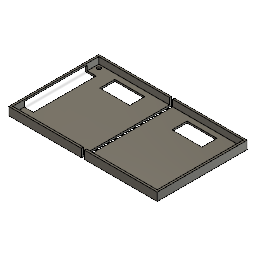
Screen_Case (Autodesk Fusion 360 design; units mm, degrees)
Autodesk Fusion 360 part; units mm, degrees
sketch "Sketch1" plane through (0, 0, 0) normal (0, 1, 0) x (1, 0, 0)
  line L0 (-122, 75.5) -> (122, 75.5)
  line L1 (122, 75.5) -> (122, -75.5)
  line L2 (122, -75.5) -> (-122, -75.5)
  line L3 (-122, -75.5) -> (-122, 75.5)
  line L4 (-122, 75.5) -> (122, -75.5) construction
  line L5 (122, 75.5) -> (-122, -75.5) construction
  dimension "d1" = 244
  dimension "d2" = 151
  constraint horizontal L0
  constraint perpendicular L0 L1
  constraint parallel L0 L2
  constraint parallel L1 L3
  constraint coincident L4 origin
  constraint coincident L5 origin
  measures "d1" distance of L1.end L2.end
  measures "d2" distance of L0.end L1.end
extrude "Extrude1" add sketch "Sketch1" along normal blind 14 makes body 1
sketch "Sketch3" plane through (0, 14, 0) normal (0, 1, 0) x (-1, 0, 0)
  line L0 (122, 75.5) -> (-122, 75.5)
  line L1 (-122, 75.5) -> (-122, -75.5)
  line L2 (-122, -75.5) -> (122, -75.5)
  line L3 (122, -75.5) -> (122, 75.5)
  line L4 (118.75, 72.25) -> (-118.75, 72.25)
  line L5 (-118.75, 72.25) -> (-118.75, -72.25)
  line L6 (-118.75, -72.25) -> (118.75, -72.25)
  line L7 (118.75, -72.25) -> (118.75, 72.25)
  line L8 (118.75, 72.25) -> (-118.75, -72.25) construction
  line L9 (-118.75, 72.25) -> (118.75, -72.25) construction
  dimension "d5" = 237.5
  dimension "d6" = 144.5
  constraint horizontal L4
  constraint perpendicular L4 L5
  constraint parallel L4 L6
  constraint parallel L5 L7
  constraint coincident L8 origin
  constraint coincident L9 origin
  measures "d5" distance of L5.end L6.end
  measures "d6" distance of L4.end L5.end
extrude "Extrude2" cut sketch "Sketch3" against normal blind 11 contours L4 L5 L6 L7 bodies 1
sketch "Sketch5" plane through (0, 5, 0) normal (0, 1, 0) x (-1, 0, 0)
  line L0 (118, -71.5) -> (118, 71.5)
  line L1 (118, 71.5) -> (-118, 71.5)
  line L2 (-118, 71.5) -> (-118, -71.5)
  line L3 (-118, -71.5) -> (118, -71.5)
  line L4 (0, 40.5) -> (-42, 40.5)
  line L5 (-42, 40.5) -> (48, 40.5)
  line L6 (48, 40.5) -> (48, -17.5)
  line L7 (48, -17.5) -> (-42, -17.5)
  line L8 (-42, -17.5) -> (-42, 40.5)
  constraint perpendicular L5 L6
  constraint perpendicular L6 L7
  constraint perpendicular L5 L8
extrude "Extrude3" [suppressed]
sketch "Sketch6" plane through (0, 3, 0) normal (0, 1, 0) x (-1, 0, 0)
  line L0 (118.75, -72.25) -> (118.75, 72.25)
  line L1 (118.75, 72.25) -> (-118.75, 72.25)
  line L2 (-118.75, 72.25) -> (-118.75, -72.25)
  line L3 (-118.75, -72.25) -> (118.75, -72.25)
  line L4 (118.75, -72.25) -> (123.75, -72.25) construction
  circle A0 centre (113, -66.5) radius 3.5
  circle A1 centre (113, 66.5) radius 3.5
  circle A2 centre (-113, 66.5) radius 3.5
  circle A3 centre (-113, -66.5) radius 3.5
  dimension "d18" = 7
  dimension "d21" = 7
  dimension "d22" = 7
  dimension "d23" = 7
  constraint horizontal L4
  constraint coincident L0.start L3.end
  measures "d18" diameter of A0
  measures "d21" diameter of A1
  measures "d22" diameter of A2
  measures "d23" diameter of A3
hole "Hole1" at (113, 3, -66.5) at (-113, 3, -66.5) at (-113, 3, 66.5) at (113, 3, 66.5) direction (0, -1, 0) diameter 6 depth 5 tip angle 180 bodies 1
sketch "Sketch7" plane through (0, 3, 0) normal (0, 1, 0) x (-1, 0, 0)
  circle A0 centre (113, 66.5) radius 3
  circle A1 centre (-113, -66.5) radius 3
  circle A2 centre (113, -66.5) radius 3
  circle A3 centre (-113, 66.5) radius 3
  line L0 (118.75, -72.25) -> (118.75, 72.25)
  line L1 (118.75, 72.25) -> (-118.75, 72.25)
  line L2 (-118.75, 72.25) -> (-118.75, -72.25)
  line L3 (-118.75, -72.25) -> (118.75, -72.25)
  line L4 (78, -63.5) -> (38, -63.5)
  line L5 (78, -63.5) -> (78, -45.5)
  line L6 (78, -45.5) -> (38, -45.5)
  line L7 (38, -45.5) -> (38, -63.5)
  line L8 (-78, -63.5) -> (-78, -45.5)
  line L9 (-78, -45.5) -> (-38, -45.5)
  line L10 (-38, -45.5) -> (-38, -63.5)
  line L11 (-38, -63.5) -> (-78, -63.5)
  line L12 (-38, -63.5) -> (-83, -63.5)
  line L13 (-83, -63.5) -> (-33, -63.5)
  line L14 (-33, -63.5) -> (-33, -38.5)
  line L15 (-33, -38.5) -> (-83, -38.5)
  line L16 (-83, -38.5) -> (-83, -63.5)
  line L17 (38, -63.5) -> (33, -63.5)
  line L18 (33, -63.5) -> (33, -38.5)
  line L19 (33, -38.5) -> (83, -38.5)
  line L20 (83, -38.5) -> (83, -63.5)
  line L21 (83, -63.5) -> (77.0132, -63.5)
  dimension "d37" = 45
  dimension "d38" = 50
  dimension "d39" = 25
  dimension "d40" = 5
  dimension "d41" = 50
  constraint perpendicular L0 L4
  constraint perpendicular L4 L5
  constraint perpendicular L5 L6
  constraint perpendicular L4 L7
  constraint perpendicular L6 L8
  constraint perpendicular L7 L9
  constraint perpendicular L4 L10
  constraint perpendicular L8 L11
  constraint perpendicular L8 L12
  constraint parallel L11 L13
  constraint perpendicular L13 L14
  constraint perpendicular L14 L15
  constraint perpendicular L13 L16
  constraint perpendicular L7 L17
  constraint perpendicular L15 L18
  constraint perpendicular L18 L19
  constraint perpendicular L19 L20
  constraint coincident L4 L21.end
  constraint perpendicular L5 L21
  measures "d37" distance of L10.end L12.end
  measures "d38" distance of L12.end L13.end
  measures "d39" distance of L13.end L14.end
  measures "d40" distance of L4.end L17.end
  measures "d41" distance of L18.end L19.end
extrude "Extrude4" cut sketch "Sketch7" against normal blind 20 contours L4 L5 L6 L7 L21 | L5 L6 L7 L17 L18 L19 L20 L21 | L8 L9 L10 L12 L13 L14 L15 L16 | L8 L9 L10 L11 L12 L13 bodies 1
split "Split1" by plane through (0, 0, 0) normal (1, 0, 0) bodies 1 makes body 2 at (47.8006, 0, 34)
move_body "Move1" bodies 2 to x (1, 0, 0) y (0, 1, 0) z (0, 0, 1) at (5, 0, 0)
sketch "Sketch8" plane through (0, 3, 0) normal (0, 1, 0) x (-1, 0, 0)
  line L0 (0, 72.25) -> (0, -72.25)
  line L1 (0, -72.25) -> (118.75, -72.25)
  line L2 (118.75, -72.25) -> (118.75, 72.25)
  line L3 (118.75, 72.25) -> (0, 72.25)
  line L4 (33, -38.5) -> (83, -38.5)
  line L5 (83, -38.5) -> (83, -63.5)
  line L6 (83, -63.5) -> (33, -63.5)
  line L7 (33, -63.5) -> (33, -38.5)
  circle A0 centre (113, 66.5) radius 3
  circle A1 centre (113, -66.5) radius 3
  line L8 (118.75, 72.25) -> (118.75, 52.25)
  line L9 (118.75, 52.25) -> (103.75, 52.25)
  line L10 (103.75, 52.25) -> (103.75, -52.75)
  line L11 (103.75, -52.75) -> (118.75, -52.75)
  line L12 (118.75, -52.75) -> (118.75, 52.25)
  dimension "d42" = 20
  dimension "d43" = 15
  dimension "d44" = 105
  constraint coincident L2.end L3.start
  constraint perpendicular L3 L8
  constraint horizontal L9
  constraint vertical L10
  constraint horizontal L11
  constraint vertical L12
  measures "d42" distance of L2.end L8.end
  measures "d43" distance of L8.end L9.end
  measures "d44" distance of L8.end L11.end
sketch "Sketch9" plane through (-118.75, 0, 0) normal (1, 0, 0) x (0, 0, -1)
  line L0 (72.25, 14) -> (-72.25, 14)
  line L1 (-72.25, 14) -> (-72.25, 3)
  line L2 (-72.25, 3) -> (72.25, 3)
  line L3 (72.25, 3) -> (72.25, 14)
  line L4 (52.75, 3) -> (-52.25, 3)
  line L5 (-52.25, 3) -> (-52.25, 11)
  line L6 (-52.25, 11) -> (52.75, 11)
  line L7 (52.75, 11) -> (52.75, 3)
  point P0 (52.75, 3)
  dimension "d45" = 8
  constraint horizontal L4
  constraint vertical L5
  constraint horizontal L6
  constraint vertical L7
  constraint coincident P0 L4.start
  measures "d45" distance of P0 L6.end
extrude "Extrude5" cut sketch "Sketch9" against normal blind 10 contours L2 L4 L5 L6 L7 bodies 1
extrude "Extrude6" cut sketch "Sketch8" against normal blind 20 contours L2 L9 L10 L11 L12 bodies 1
sketch "Sketch10" plane through (0, 3, 0) normal (0, 1, 0) x (-1, 0, 0)
  line L0 (118.75, 52.25) -> (118.75, -52.75)
  line L1 (118.75, -52.75) -> (122, -52.75)
  line L2 (122, -52.75) -> (122, 52.25)
  line L3 (122, 52.25) -> (118.75, 52.25)
  line L4 (122, 52.25) -> (118.75, 52.25)
  line L5 (118.75, 52.25) -> (118.75, -52.75)
  line L6 (118.75, -52.75) -> (122, -52.75)
  line L7 (122, -52.75) -> (122, 52.25)
  constraint horizontal L4
  constraint vertical L5
  constraint horizontal L6
  constraint vertical L7
  constraint coincident L0.end L1.start
  constraint coincident L2.end L3.start
extrude "Extrude7" cut sketch "Sketch10" against normal blind 15 bodies 1
equation "d1 = 236 mm + 8 mm"
equation "d2 = 143 mm + 8 mm"
equation "d5 = 236 mm + 1.5 mm"
equation "d6 = 143 mm + 1.5 mm"
equation "d45 = 11 mm - 3 mm"
